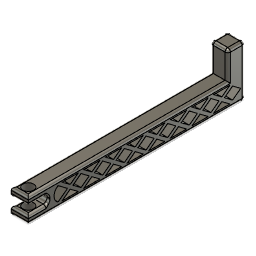
SliderPart (Autodesk Fusion 360 design; units mm, degrees)
Autodesk Fusion 360 part; units mm, degrees
sketch "Sketch1" plane through (0, 0, 38.0598) normal (0, 0, -1) x (-1, 0, 0)
  line L0 (3.3454, -62.9838) -> (3.3454, -50.9838)
  line L1 (3.3454, -50.9838) -> (1.3454, -50.9838)
  line L2 (1.3454, -50.7342) -> (-1.4546, -50.7342)
  line L3 (-1.4546, -50.9838) -> (-3.4546, -50.9838)
  line L4 (-3.4546, -50.9838) -> (-3.4546, -62.9838)
  arc A0 (-3.4546, -62.9838) -> (-2.4546, -63.9838) centre (-2.4546, -62.9838) ccw
  line L5 (-2.4546, -63.9838) -> (2.3454, -63.9838)
  arc A1 (2.3454, -63.9838) -> (3.3454, -62.9838) centre (2.3454, -62.9838) ccw
  line L6 (-3.3046, -62.9838) -> (-3.3046, -52.9838)
  line L7 (-3.3046, -52.9838) -> (3.1954, -52.9838)
  line L8 (3.1954, -52.9838) -> (3.1954, -62.9838)
  line L9 (3.1954, -62.9838) -> (-3.3046, -62.9838)
  line L10 (-0.0546, -52.9838) -> (3.0954, -52.9838)
  line L11 (3.0954, -52.9838) -> (3.0954, -61.9838)
  line L12 (-0.0546, -52.9838) -> (-3.2046, -52.9838)
  line L13 (-3.2046, -52.9838) -> (3.0954, -52.9838)
  line L14 (3.0954, -52.9838) -> (3.0954, -61.9838)
  line L15 (3.0954, -61.9838) -> (-3.2046, -61.9838)
  line L16 (-3.2046, -61.9838) -> (-3.2046, -52.9838)
  line L17 (1.3454, -50.9838) -> (1.3454, -50.7342)
  line L18 (-1.4546, -50.7342) -> (-1.4546, -50.9838)
  dimension "d252" = 3.15
  dimension "d253" = 9
  dimension "d254" = 3.15
  constraint midpoint L7 L10.start
  constraint parallel L7 L10
  constraint perpendicular L10 L11
  constraint perpendicular L8 L12
  constraint horizontal L13
  constraint vertical L14
  constraint horizontal L15
  constraint vertical L16
  measures "d252" distance of L10.start L10.end
  measures "d253" distance of L10.end L11.end
  measures "d254" distance of L10.start L12.end
extrude "Extrude1" add sketch "Sketch1" against normal blind 50 contours L7 L10 L11 L12 L13 L14 L15 L16
extrude "Extrude2" add 1 faces at (0.0546, -58.9838, 38.0598) along direction (0, 0, -1) blind 30
sketch "Sketch2" plane through (0, -52.9838, 0) normal (0, 1, 0) x (-1, 0, 0)
  line L0 (3.0954, 8.0598) -> (3.0954, 88.0598)
  line L1 (3.0954, 88.0598) -> (-3.2046, 88.0598)
  line L2 (-3.2046, 88.0598) -> (-3.2046, 8.0598)
  line L3 (-3.2046, 8.0598) -> (3.0954, 8.0598)
  line L4 (3.0954, 8.0598) -> (-3.2046, 8.0598)
  line L5 (-3.2046, 8.0598) -> (-3.2046, 14.3598)
  line L6 (-3.2046, 14.3598) -> (3.0954, 14.3598)
  line L7 (3.0954, 14.3598) -> (3.0954, 8.0598)
  dimension "d259" = 6.3
  constraint horizontal L4
  constraint vertical L5
  constraint horizontal L6
  constraint vertical L7
  constraint coincident L0.start L3.end
  measures "d259" distance of L0.start L6.end
extrude "Extrude3" add sketch "Sketch2" along normal blind 10 contours L0 L2 L3 L4 L5 L6 L7
sketch "Sketch3" plane through (0, -52.9838, 0) normal (0, 1, 0) x (-1, 0, 0)
  line L0 (-3.2046, 14.3598) -> (3.0954, 14.3598)
  line L1 (3.0954, 14.3598) -> (3.0954, 88.0598)
  line L2 (3.0954, 88.0598) -> (-3.2046, 88.0598)
  line L3 (-3.2046, 88.0598) -> (-3.2046, 14.3598)
  line L4 (-0.0546, 88.0598) -> (-0.0546, 84.9098)
  circle A0 centre (-0.0546, 84.9098) radius 2
  dimension "d262" = 3.15
  dimension "d263" = 4
  constraint midpoint L2 L4.start
  constraint perpendicular L2 L4
  constraint coincident L4.end A0.centre
  measures "d262" distance of L4.start L4.end
  measures "d263" diameter of A0
extrude "Extrude4" cut sketch "Sketch3" against normal blind 13.5 contours A0
sketch "Sketch4" plane through (0, 0, 88.0598) normal (0, 0, 1) x (1, 0, 0)
  line L0 (-3.0954, -61.9838) -> (3.2046, -61.9838)
  line L1 (3.2046, -61.9838) -> (3.2046, -52.9838)
  line L2 (3.2046, -52.9838) -> (-3.0954, -52.9838)
  line L3 (-3.0954, -52.9838) -> (-3.0954, -61.9838)
  line L4 (3.2046, -57.4838) -> (3.2046, -55.9838)
  line L5 (3.2046, -55.9838) -> (-3.0954, -55.9838)
  line L6 (-3.0954, -55.9838) -> (-3.0954, -58.9838)
  line L7 (-3.0954, -58.9838) -> (3.2046, -58.9838)
  line L8 (3.2046, -58.9838) -> (3.2046, -55.9838)
  dimension "d266" = 1.5
  dimension "d267" = 3
  constraint midpoint L1 L4.start
  constraint perpendicular L2 L4
  constraint horizontal L5
  constraint vertical L6
  constraint horizontal L7
  constraint vertical L8
  measures "d266" distance of L4.start L4.end
  measures "d267" distance of L4.end L7.end
extrude "Extrude5" cut sketch "Sketch4" against normal blind 8 contours L1 L3 L4 L5 L6 L7 L8
sketch "Sketch5" plane through (3.2046, 0, 0) normal (1, 0, 0) x (0, 0, -1)
  line L0 (-88.0598, -55.9838) -> (-80.0598, -55.9838)
  line L1 (-80.0598, -55.9838) -> (-80.0598, -58.9838)
  line L2 (-80.0598, -58.9838) -> (-88.0598, -58.9838)
  line L3 (-88.0598, -58.9838) -> (-88.0598, -61.9838)
  line L4 (-88.0598, -61.9838) -> (-8.0598, -61.9838)
  line L5 (-8.0598, -61.9838) -> (-8.0598, -42.9838)
  line L6 (-8.0598, -42.9838) -> (-14.3598, -42.9838)
  line L7 (-14.3598, -42.9838) -> (-14.3598, -52.9838)
  line L8 (-14.3598, -52.9838) -> (-88.0598, -52.9838)
  line L9 (-88.0598, -52.9838) -> (-88.0598, -55.9838)
  line L10 (-80.0598, -57.4838) -> (-75.5598, -57.4838)
  circle A0 centre (-75.5598, -57.4838) radius 3
  line L11 (-14.3598, -52.9838) -> (-8.0598, -52.9838)
  line L12 (-8.0598, -52.9838) -> (-8.0598, -61.9838)
  line L13 (-8.0598, -57.4838) -> (-12.5598, -57.4838)
  circle A1 centre (-12.5598, -57.4838) radius 3
  line L14 (-12.5598, -60.4828) -> (-12.5598, -54.4838)
  line L15 (-75.5598, -57.4838) -> (-75.5598, -54.4838)
  line L16 (-75.5598, -57.4838) -> (-75.5598, -60.4838)
  line L17 (-75.5598, -60.4838) -> (-12.5598, -60.4828)
  line L18 (-12.5598, -54.4838) -> (-75.5598, -54.4838)
  dimension "d270" = 4.5
  dimension "d272" = 4.5
  dimension "d273" = 6
  constraint midpoint L1 L10.start
  constraint perpendicular L1 L10
  constraint coincident L10.end A0.centre
  constraint coincident L7.end L8.start
  constraint coincident L5 L11.end
  constraint perpendicular L5 L11
  constraint coincident L4 L5.start
  constraint coincident L5 L4.end
  constraint midpoint L12 L13.start
  constraint perpendicular L12 L13
  constraint coincident L13.end A1.centre
  constraint vertical L14
  constraint coincident A1 L14.end
  constraint coincident A0 L15.end
  constraint perpendicular L10 L15
  constraint coincident A0 L16.end
  constraint perpendicular L10 L16
  constraint tangent A0 L18
  measures "d270" distance of L10.start L10.end
  measures "d272" distance of L13.start L13.end
  measures "d273" diameter of A1
extrude "Extrude6" cut sketch "Sketch5" against normal blind 6.3 contours L10 A0 L15 | L10 A0 L16 | A0 L15 L16 | A0 A1 L17 L18 | A1 L14 | L13 A1 L14 | L13 A1 L14
sketch "Sketch6" plane through (3.2046, 0, 0) normal (1, 0, 0) x (0, 0, -1)
  arc A0 (-12.634, -60.4828) -> (-12.5598, -54.4838) centre (-12.5598, -57.4838) ccw
  arc A1 (-75.5598, -54.4838) -> (-75.5598, -60.4838) centre (-75.5598, -57.4838) ccw
  line L0 (-88.0598, -55.9838) -> (-80.0598, -55.9838)
  line L1 (-80.0598, -55.9838) -> (-80.0598, -58.9838)
  line L2 (-80.0598, -58.9838) -> (-88.0598, -58.9838)
  line L3 (-88.0598, -58.9838) -> (-88.0598, -61.9838)
  line L4 (-88.0598, -61.9838) -> (-8.0598, -61.9838)
  line L5 (-8.0598, -61.9838) -> (-8.0598, -42.9838)
  line L6 (-8.0598, -42.9838) -> (-14.3598, -42.9838)
  line L7 (-14.3598, -42.9838) -> (-14.3598, -52.9838)
  line L8 (-14.3598, -52.9838) -> (-88.0598, -52.9838)
  line L9 (-88.0598, -52.9838) -> (-88.0598, -55.9838)
  line L10 (-12.634, -60.4828) -> (-75.5598, -60.4838)
  line L11 (-75.5598, -54.4838) -> (-12.5598, -54.4838)
  line L12 (-75.5598, -60.4838) -> (-77.5598, -60.4838)
  line L13 (-75.5598, -54.4838) -> (-77.5598, -54.4838)
  line L14 (-75.5598, -54.4838) -> (-69.5598, -54.4838)
  line L15 (-69.5598, -54.4838) -> (-67.5598, -54.4838)
  line L16 (-75.5598, -60.4838) -> (-69.5598, -60.4837)
  line L17 (-69.5598, -60.4837) -> (-67.5598, -60.4836)
  line L18 (-75.5598, -54.4838) -> (-67.5598, -60.4836)
  line L19 (-69.5598, -60.4837) -> (-77.5598, -54.4838)
  line L20 (-69.5598, -54.4838) -> (-77.5598, -60.4838)
  line L21 (-75.5598, -60.4838) -> (-67.5598, -54.4838)
  line L22 (-61.5598, -60.4837) -> (-69.5598, -54.4838)
  line L23 (-67.5598, -54.4838) -> (-59.5598, -60.4836)
  line L24 (-61.5598, -54.4838) -> (-69.5598, -60.4838)
  line L25 (-67.5598, -60.4838) -> (-59.5598, -54.4838)
  line L26 (-53.5598, -60.4837) -> (-61.5598, -54.4838)
  line L27 (-59.5598, -54.4838) -> (-51.5598, -60.4836)
  line L28 (-53.5598, -54.4838) -> (-61.5598, -60.4838)
  line L29 (-59.5598, -60.4838) -> (-51.5598, -54.4838)
  line L30 (-45.5598, -60.4837) -> (-53.5598, -54.4838)
  line L31 (-51.5598, -54.4838) -> (-43.5598, -60.4836)
  line L32 (-45.5598, -54.4838) -> (-53.5598, -60.4838)
  line L33 (-51.5598, -60.4838) -> (-43.5598, -54.4838)
  line L34 (-37.5598, -60.4837) -> (-45.5598, -54.4838)
  line L35 (-43.5598, -54.4838) -> (-35.5598, -60.4836)
  line L36 (-37.5598, -54.4838) -> (-45.5598, -60.4838)
  line L37 (-43.5598, -60.4838) -> (-35.5598, -54.4838)
  line L38 (-29.5598, -60.4837) -> (-37.5598, -54.4838)
  line L39 (-35.5598, -54.4838) -> (-27.5598, -60.4836)
  line L40 (-29.5598, -54.4838) -> (-37.5598, -60.4838)
  line L41 (-35.5598, -60.4838) -> (-27.5598, -54.4838)
  line L42 (-21.5598, -60.4837) -> (-29.5598, -54.4838)
  line L43 (-27.5598, -54.4838) -> (-19.5598, -60.4836)
  line L44 (-21.5598, -54.4838) -> (-29.5598, -60.4838)
  line L45 (-27.5598, -60.4838) -> (-19.5598, -54.4838)
  line L46 (-13.5598, -60.4837) -> (-21.5598, -54.4838)
  line L47 (-19.5598, -54.4838) -> (-11.5598, -60.4836)
  line L48 (-13.5598, -54.4838) -> (-21.5598, -60.4838)
  line L49 (-19.5598, -60.4838) -> (-11.5598, -54.4838)
  line L50 (-5.5598, -60.4837) -> (-13.5598, -54.4838)
  line L51 (-11.5598, -54.4838) -> (-3.5598, -60.4836)
  line L52 (-5.5598, -54.4838) -> (-13.5598, -60.4838)
  line L53 (-11.5598, -60.4838) -> (-3.5598, -54.4838)
  dimension "d362" = 2
  dimension "d363" = 2
  dimension "d364" = 6
  dimension "d365" = 2
  dimension "d366" = 6
  dimension "d367" = 2
  dimension "d370" = 8
  dimension "d371" = 0
  constraint coincident A1.end L10.end
  constraint parallel L10 L12
  constraint coincident A1.start L11.start
  constraint parallel L11 L13
  constraint parallel L11 L14
  constraint parallel L11 L15
  constraint parallel L10 L16
  constraint parallel L10 L17
  measures "d362" distance of A1.end L12.end
  measures "d363" distance of A1.start L13.end
  measures "d364" distance of A1.start L14.end
  measures "d365" distance of L14.end L15.end
  measures "d366" distance of A1.end L16.end
  measures "d367" distance of L16.end L17.end
extrude "Extrude7" add sketch "Sketch6" against normal blind 6.3 contours A0 L10 L47 L52 | A0 L47 L52 | L46 L47 L49 L52 | L10 L43 L48 | L43 L46 L48 L49 | L46 L47 L48 L49 | A0 L49 L50 | L47 L48 L49 L50 | L42 L43 L45 L48 | L45 L46 L47 L48 | A0 L11 L49 L50 | L10 L39 L44 | L39 L42 L44 L45 | L42 L43 L44 L45 | L43 L44 L45 L46 | L11 L45 L46 | L38 L39 L41 L44 | L41 L42 L43 L44 | L10 L35 L40 | L35 L38 L40 L41 | L38 L39 L40 L41 | L39 L40 L41 L42 | L11 L41 L42 | L34 L35 L37 L40 | L37 L38 L39 L40 | L10 L31 L36 | L31 L34 L36 L37 | L34 L35 L36 L37 | L35 L36 L37 L38 | L11 L37 L38 | L30 L31 L33 L36 | L33 L34 L35 L36 | L10 L27 L32 | L27 L30 L32 L33 | L30 L31 L32 L33 | L31 L32 L33 L34 | L11 L33 L34 | L26 L27 L29 L32 | L29 L30 L31 L32 | L10 L23 L28 | L23 L26 L28 L29 | L26 L27 L28 L29 | L27 L28 L29 L30 | L11 L29 L30 | L22 L23 L25 L28 | L25 L26 L27 L28 | L10 L17 L18 L24 | L18 L22 L24 L25 | L22 L23 L24 L25 | L23 L24 L25 L26 | L11 L25 L26 | L18 L19 L21 L24 | L21 L22 L23 L24 | A1 L19 L20 L21 | L18 L19 L20 L21 | L18 L20 L21 L22 | L11 L15 L21 L22 | A1 L18 L19 L20
fillet "Fillet1" radius 1 15 edges at (3.2046, -52.9838, 51.2098) (0.0546, -52.9838, 88.0598) (-3.0954, -52.9838, 51.2098) (3.2046, -61.9838, 48.0598) (0.0546, -61.9838, 88.0598) (-3.0954, -61.9838, 48.0598) (0.0546, -61.9838, 8.0598) (3.2046, -47.9838, 14.3598) (3.2046, -52.4838, 8.0598) (-3.0954, -52.4838, 8.0598) (-3.0954, -47.9838, 14.3598) (-3.0954, -42.9838, 11.2098) (0.0546, -42.9838, 14.3598) (3.2046, -42.9838, 11.2098) (0.0546, -42.9838, 8.0598)
fillet "Fillet2" radius 1 6 edges at (0.0546, -55.9838, 88.0598) (-3.0954, -55.9838, 84.0598) (3.2046, -55.9838, 84.0598) (-3.0954, -58.9838, 84.0598) (0.0546, -58.9838, 88.0598) (3.2046, -58.9838, 84.0598)
fillet "Fillet3" radius 1.5 6 edges at (2.9117, -59.2767, 80.0598) (0.0546, -58.9838, 80.0598) (-2.8025, -59.2767, 80.0598) (-2.8025, -55.6909, 80.0598) (0.0546, -55.9838, 80.0598) (2.9117, -55.6909, 80.0598)
equation "d252 = ( 6.3 / 2 ) * 1 mm"
